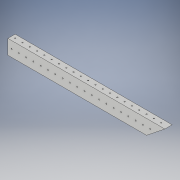
# Autodesk Inventor part: Kermit Frame1
Saved by Autodesk Inventor 2018 (Build 220112000, 112)
## iProperties
Created: 2018-02-01
Part Number: Kermit Frame1
Material: Generic
Document SubType Name: Modeling
Designer: lopez.xavier
Density: 1 g/cm^3
Appearance: Default
Author: lopez.xavier
Autodesk Inventor part; units mm, degrees
ref_plane "YZ Plane" through (0, 0, 0) normal (1, 0, 0) x (0, 1, 0)
ref_plane "XZ Plane" through (0, 0, 0) normal (0, 1, 0) x (-1, 0, 0)
ref_plane "XY Plane" through (0, 0, 0) normal (0, 0, 1) x (1, 0, 0)
sketch "Sketch1" plane through (0, 0, 0) normal (0, 0, 1) x (1, 0, 0)
  line L0 (0, 0) -> (546.1, 0)
  line L1 (546.1, 0) -> (546.1, 50.8)
  line L2 (546.1, 50.8) -> (0, 50.8)
  line L3 (0, 50.8) -> (0, 0)
  dimension "d0" = 546.1
  dimension "d1" = 50.8
  constraints: 8 end point, 2 parallel, 1 horizontal, 1 perpendicular
  measures "d0" distance of L1.end L2.end
  measures "d1" distance of L0.end L1.end
extrude "Extrusion1" add sketch "Sketch1" along normal blind 25.4
sketch "Sketch2" plane through (0, 0, 25.4) normal (0, 0, 1) x (1, 0, 0)
  line L0 (0, 0) -> (546.1, 0) projected
  line L1 (546.1, 0) -> (546.1, 50.8) projected
  line L2 (482.6, 0) -> (546.1, 50.8)
  line L3 (482.6, 0) -> (546.1, 0)
  line L4 (546.1, 0) -> (546.1, 50.8)
  dimension "d4" = 63.5
  constraints: 6 end point, 1 horizontal, 1 perpendicular, 1 point on line
  measures "d4" distance of L0.end L2.start
extrude "Extrusion2" cut sketch "Sketch2" against normal blind 25.4
sketch "Sketch3" plane through (0, 0, 0) normal (-1, 0, 0) x (0, 0, 1)
  line L0 (3.175, 47.625) -> (22.225, 47.625)
  line L1 (22.225, 47.625) -> (22.225, 3.175)
  line L2 (22.225, 3.175) -> (3.175, 3.175)
  line L3 (3.175, 3.175) -> (3.175, 47.625)
  line L4 (25.4, 50.8) -> (25.4, 0) projected
  line L5 (0, 50.8) -> (25.4, 50.8) projected
  line L6 (0, 0) -> (25.4, 0) projected
  line L7 (0, 50.8) -> (0, 0) projected
  dimension "d7" = 3.175
  dimension "d8" = 3.175
  dimension "d9" = 3.175
  dimension "d10" = 3.175
  constraints: 8 end point, 2 parallel, 1 horizontal, 1 perpendicular
  measures "d7" distance between parallel lines of L4 L1
  measures "d8" distance between parallel lines of L5 L0
  measures "d9" distance between parallel lines of L6 L2
  measures "d10" distance between parallel lines of L7 L3
extrude "Extrusion3" cut sketch "Sketch3" against normal blind 635 contours L0 L1 L2 L3
sketch "Sketch4" plane through (0, 0, 25.4) normal (0, 0, 1) x (1, 0, 0)
  circle A0 centre (12.7, 25.4) radius 1.9685
  line L0 (546.1, 50.8) -> (0, 50.8) projected
  line L1 (0, 50.8) -> (0, 0) projected
  circle A1 centre (38.1, 25.4) radius 1.9685
  circle A2 centre (63.5, 25.4) radius 1.9685
  circle A3 centre (88.9, 25.4) radius 1.9685
  circle A4 centre (114.3, 25.4) radius 1.9685
  circle A5 centre (139.7, 25.4) radius 1.9685
  circle A6 centre (165.1, 25.4) radius 1.9685
  circle A7 centre (190.5, 25.4) radius 1.9685
  circle A8 centre (215.9, 25.4) radius 1.9685
  circle A9 centre (241.3, 25.4) radius 1.9685
  circle A10 centre (266.7, 25.4) radius 1.9685
  circle A11 centre (292.1, 25.4) radius 1.9685
  circle A12 centre (317.5, 25.4) radius 1.9685
  circle A13 centre (342.9, 25.4) radius 1.9685
  circle A14 centre (368.3, 25.4) radius 1.9685
  circle A15 centre (393.7, 25.4) radius 1.9685
  circle A16 centre (419.1, 25.4) radius 1.9685
  circle A17 centre (444.5, 25.4) radius 1.9685
  circle A18 centre (469.9, 25.4) radius 1.9685
  circle A19 centre (495.3, 25.4) radius 1.9685
  dimension "d13" = 3.937
  dimension "d14" = 25.4
  dimension "d15" = 12.7
  dimension "d18" = 25.4
  constraints: 20 centre point, 1 horizontal, 38 other
  measures "d13" diameter of A0
  measures "d14" distance from line of L0 A0.centre
  measures "d15" distance from line of L1 A0.centre
  measures "d18" distance of A0.centre A1.centre
extrude "Extrusion4" cut sketch "Sketch4" against normal blind 254
sketch "Sketch5" plane through (0, 50.8, 25.4) normal (0, 1, 0) x (1, 0, 0)
  circle A0 centre (12.7, 12.7) radius 1.9685
  line L0 (546.1, 0) -> (0, 0) projected
  line L1 (0, 25.4) -> (0, 0) projected
  circle A1 centre (38.1, 12.7) radius 1.9685
  circle A2 centre (63.5, 12.7) radius 1.9685
  circle A3 centre (88.9, 12.7) radius 1.9685
  circle A4 centre (114.3, 12.7) radius 1.9685
  circle A5 centre (139.7, 12.7) radius 1.9685
  circle A6 centre (165.1, 12.7) radius 1.9685
  circle A7 centre (190.5, 12.7) radius 1.9685
  circle A8 centre (215.9, 12.7) radius 1.9685
  circle A9 centre (241.3, 12.7) radius 1.9685
  circle A10 centre (266.7, 12.7) radius 1.9685
  circle A11 centre (292.1, 12.7) radius 1.9685
  circle A12 centre (317.5, 12.7) radius 1.9685
  circle A13 centre (342.9, 12.7) radius 1.9685
  circle A14 centre (368.3, 12.7) radius 1.9685
  circle A15 centre (393.7, 12.7) radius 1.9685
  circle A16 centre (419.1, 12.7) radius 1.9685
  circle A17 centre (444.5, 12.7) radius 1.9685
  circle A18 centre (469.9, 12.7) radius 1.9685
  circle A19 centre (495.3, 12.7) radius 1.9685
  circle A20 centre (520.7, 12.7) radius 1.9685
  dimension "d25" = 3.937
  dimension "d26" = 12.7
  dimension "d27" = 12.7
  dimension "d30" = 25.4
  constraints: 21 centre point, 1 horizontal, 40 other
  measures "d25" diameter of A0
  measures "d26" distance from line of L0 A0.centre
  measures "d27" distance from line of L1 A0.centre
  measures "d30" distance of A0.centre A1.centre
extrude "Extrusion5" cut sketch "Sketch5" against normal blind 254
body "Solid1"
